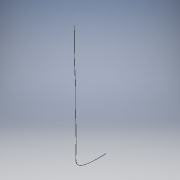
# Autodesk Inventor part: PowerCable
Saved by Autodesk Inventor 2017 (Build 210142000, 142)
## iProperties
Created: 2017-10-10
Part Number: PowerCable
Material: Generic
Document SubType Name: Modeling
Designer: Kathryn Rosie
Density: 1 g/cm^3
Appearance: Generic
Author: Kathryn Rosie
Autodesk Inventor part; units mm, degrees
ref_plane "YZ Plane" through (0, 0, 0) normal (1, 0, 0) x (0, 1, 0)
ref_plane "XZ Plane" through (0, 0, 0) normal (0, 1, 0) x (-1, 0, 0)
ref_plane "XY Plane" through (0, 0, 0) normal (0, 0, 1) x (1, 0, 0)
sketch "Sketch1" plane through (0, 0, 0) normal (1, 0, 0) x (0, 1, 0)
  line L0 (-41.6909, 2719.5207) -> (-67.8675, 1907.4512) construction
  line L1 (-67.8675, 1907.4512) -> (-6.5285, 563.5042) construction
  line L2 (-6.5285, 563.5042) -> (-6.5285, 324.5897) construction
  line L3 (-6.5285, 324.5897) -> (14.9092, 13.411) construction
  line L4 (14.9092, 13.411) -> (-12.8137, -511.0804) construction
  line L5 (-12.8137, -511.0804) -> (58.4562, -2016.5581) construction
  line L6 (58.4562, -2016.5581) -> (17.8661, -2736.3946) construction
  line L7 (17.8661, -2736.3946) -> (-12.8137, -3280.4793) construction
  line L8 (-12.8137, -3280.4793) -> (1433.5397, -3227.5942) construction
  spline S0 degree 4 poles (-41.6909, 2719.5207) (-67.8675, 1907.4512) (-6.5285, 563.5042) (-6.5285, 324.5897) (14.9092, 13.411) (-12.8137, -511.0804) (58.4562, -2016.5581) (17.8661, -2736.3946) (-12.8137, -3280.4793) (1433.5397, -3227.5942) knots 1 1 1 1 1 2 3 4 5 6 7 7 7 7 7
  point P0 (0, 0)
  dimension "d1" = 6000
  constraints: 3 other
  measures "d1" vertical distance of L7.end L0.start
sketch "Sketch2" plane through (0, 0, 0) normal (0, 0, 1) x (1, 0, 0)
  circle A0 centre (0, 0) radius 8
  dimension "d0" = 16
  constraints: 1 centre point, 1 coincident
  measures "d0" diameter of A0
sweep "Sweep1" add profiles "Sketch2" path "Sketch1"
body "Solid1"
